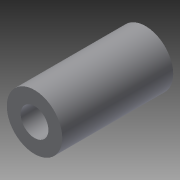
# Autodesk Inventor part: Servo Mount
Saved by Autodesk Inventor 2014 SP1 (Build 180222100, 222)
## iProperties
Created: 2014-01-26
Part Number: Servo Mount
Material: Generic
Document SubType Name: Modeling
Designer: tom
Density: 1 g/cm^3
Appearance: Default
Author: tom
Autodesk Inventor part; units mm, degrees
ref_plane "YZ Plane" through (0, 0, 0) normal (1, 0, 0) x (0, 1, 0)
ref_plane "XZ Plane" through (0, 0, 0) normal (0, 1, 0) x (-1, 0, 0)
ref_plane "XY Plane" through (0, 0, 0) normal (0, 0, 1) x (1, 0, 0)
sketch "Sketch1" plane through (0, 0, 0) normal (0, 0, 1) x (1, 0, 0)
  circle A0 centre (0, 0) radius 3.175
  circle A1 centre (0, 0) radius 6.35
  line L0 (-9.9825, 5.08) -> (3.81, 5.08) construction
  line L1 (-9.9825, -3.81) -> (5.08, -3.81) construction
  line L2 (-9.9825, 6.89) -> (5.08, 6.89) construction
  line L3 (-6.35, 0) -> (-6.35, 11.89) construction
  line L4 (-12.6478, 11.89) -> (5.5321, 11.89) construction
  line L5 (-3.35, 11.89) -> (-3.35, 6.89) construction
  line L6 (-3.35, 11.89) -> (4.3574, 4.619)
  line L7 (-6.35, 0) -> (-6.35, 6.89)
  line L8 (-6.35, 11.89) -> (-26.416, 11.89)
  line L9 (-26.416, 11.89) -> (-31.416, 11.89)
  line L10 (-31.416, 11.89) -> (-31.416, 6.89)
  line L11 (-31.416, 6.89) -> (-6.35, 6.89)
  line L12 (-6.35, 11.89) -> (-3.35, 11.89)
  dimension "d0" = 6.35
  dimension "d1" = 12.7
  dimension "d4" = 5.08
  dimension "d5" = 3.81
  dimension "d7" = 5
  dimension "d8" = 3
  dimension "d9" = 20.066
  dimension "d10" = 5
  dimension "d11" = 11.89
  constraints: 26 end point, 5 perpendicular, 5 point on line, 4 parallel, 4 point on circle, 2 centre point, 2 coincident, 2 tangent, 1 collinear
  measures "d0" diameter of A0
  measures "d1" diameter of A1
  measures "d4" distance from line of L0 point (0, 0)
  measures "d5" distance from line of L1 point (0, 0)
  measures "d7" distance between parallel lines of L4 L2
  measures "d8" distance between parallel lines of L5 L3
  measures "d9" distance of L3.end L8.end
  measures "d10" distance of L8.end L9.end
  measures "d11" distance from line of point (0, 0) L8
extrude "Extrusion1" add sketch "Sketch1" against normal blind 25.4
sketch "Sketch2" plane through (0, 0, 0) normal (0, 0, 1) x (1, 0, 0)
  line L0 (-31.416, 11.89) -> (-31.416, 6.89) projected
  line L1 (-6.35, 6.89) -> (-6.35, 0) projected
  line L2 (-3.35, 11.89) -> (-3.35, 6.89)
  line L3 (-3.35, 6.89) -> (-31.416, 6.89)
  line L4 (-31.416, 11.89) -> (-3.35, 11.89)
  constraints: 6 end point, 2 parallel, 1 perpendicular
extrude "Extrusion2" add sketch "Sketch2" along normal blind 26.416
sketch "Sketch3" plane through (-31.416, 6.89, -25.4) normal (0, -1, 0) x (1, 0, 0)
  line L0 (0, 0) -> (0, 51.816) projected
  line L1 (25.066, 0) -> (0, 0) projected
  line L2 (25.066, 25.4) -> (25.066, 0) projected
  line L3 (0, 51.816) -> (28.066, 51.816) projected
  line L4 (5, 5) -> (25.066, 5)
  line L5 (5, 5) -> (5, 46.816)
  line L6 (5, 46.816) -> (25.066, 46.816)
  line L7 (25.066, 46.816) -> (25.066, 5)
  point P0 (31.416, 25.4)
  dimension "d14" = 5
  dimension "d15" = 5
  dimension "d16" = 5
  constraints: 8 end point, 2 perpendicular, 1 parallel, 1 point on line
  measures "d14" distance between parallel lines of L4 L1
  measures "d15" distance between parallel lines of L0 L5
  measures "d16" distance between parallel lines of L3 L6
extrude "Extrusion3" cut sketch "Sketch3" against normal blind 5
move faces "Move Face1" translate (0, -2, 0) faces at (-29.7493, 6.89, 7.4773)
sketch "Sketch5" plane through (-31.416, 4.89, 26.416) normal (0, -1, 0) x (1, 0, 0)
  line L0 (5, -5) -> (25.066, -5) projected
  line L1 (28.066, -26.416) -> (28.066, 0) projected
  line L2 (0, 0) -> (28.066, 0) projected
  line L3 (0, -51.816) -> (0, 0) projected
  line L4 (15.033, -5) -> (15.033, 0) construction
  line L5 (9.953, -3) -> (9.953, 0) construction
  line L6 (20.113, -5) -> (20.113, 0) construction
  line L7 (0, -3) -> (28.066, -3) construction
  circle A0 centre (9.953, -1.5) radius 2.375
  line L8 (9.953, -1.5) -> (20.113, -1.5) construction
  circle A1 centre (20.113, -1.5) radius 2.25
  line L9 (25.066, -46.816) -> (25.066, -51.816) projected
  line L10 (0, -25.908) -> (28.066, -25.908) construction
  circle A2 centre (9.953, -50.316) radius 2.375
  circle A3 centre (20.113, -50.316) radius 2.25
  point P0 (31.416, -26.416)
  dimension "d25" = 5.08
  dimension "d26" = 5.08
  dimension "d27" = 2
  dimension "d28" = 4.75
  dimension "d30" = 4.5
  constraints: 12 end point, 9 point on line, 4 centre point, 4 perpendicular, 3 midpoint, 2 parallel, 2 symmetric about line, 1 coincident, 2 other
  measures "d25" distance between parallel lines of L5 L4
  measures "d26" distance between parallel lines of L4 L6
  measures "d27" distance between parallel lines of L7 L0
  measures "d28" diameter of A0
  measures "d30" diameter of A1
extrude "Extrusion5" cut sketch "Sketch5" against normal blind 7
chamfer "Chamfer1" distance 2 angle 45 3 edges at (-31.416, 8.39, 26.416) (-31.416, 8.39, -25.4) (-3.35, 8.39, 26.416)
body "Solid1"
